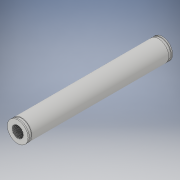
# Autodesk Inventor part: Axel_SBail
Saved by Autodesk Inventor 2019 (Build 230136000, 136)
## iProperties
Created: 2019-04-10
Part Number: Axel_SBail
Material: Generic
Document SubType Name: Modeling
Designer: samson.bailor
Density: 1 g/cm^3
Appearance: Default
Author: samson.bailor
Autodesk Inventor part; units mm, degrees
ref_plane "YZ Plane" through (0, 0, 0) normal (1, 0, 0) x (0, 1, 0)
ref_plane "XZ Plane" through (0, 0, 0) normal (0, 1, 0) x (-1, 0, 0)
ref_plane "XY Plane" through (0, 0, 0) normal (0, 0, 1) x (1, 0, 0)
sketch "Sketch1" plane through (0, 0, 0) normal (0, 0, 1) x (1, 0, 0)
  circle A0 centre (0, 0) radius 25.4
  dimension "d0" = 50.8
  constraints: 1 centre point, 1 coincident
  measures "d0" diameter of A0
extrude "Extrusion1" add sketch "Sketch1" along normal blind 355.6
sketch "Sketch2" plane through (0, 0, 355.6) normal (0, 0, 1) x (1, 0, 0)
  line L0 (0, 13.97) -> (0.508, 13.97)
  line L1 (0, 13.97) -> (-0.508, 13.97)
  line L2 (-0.508, 13.97) -> (-0.856, 12.6711)
  line L3 (-0.508, 13.97) -> (1.4308, 13.97) construction
  line L4 (0.508, 13.97) -> (0.856, 12.6711)
  line L5 (0.508, 13.97) -> (2.6446, 13.97) construction
  line L6 (-2.4076, 13.7703) -> (-1.7971, 12.5722)
  line L7 (-3.4014, 13.5591) -> (-3.4718, 12.2162)
  line L8 (-2.9045, 13.6647) -> (-3.4014, 13.5591)
  line L9 (-2.9045, 13.6647) -> (-2.4076, 13.7703)
  line L10 (-5.218, 12.9689) -> (-4.3718, 11.9238)
  line L11 (-6.1462, 12.5556) -> (-5.9358, 11.2275)
  line L12 (-5.6821, 12.7622) -> (-6.1462, 12.5556)
  line L13 (-5.6821, 12.7622) -> (-5.218, 12.9689)
  line L14 (-7.8004, 11.6006) -> (-6.7553, 10.7543)
  line L15 (-8.6223, 11.0034) -> (-8.1404, 9.748)
  line L16 (-8.2114, 11.302) -> (-8.6223, 11.0034)
  line L17 (-8.2114, 11.302) -> (-7.8004, 11.6006)
  line L18 (-10.0418, 9.7253) -> (-8.8437, 9.1148)
  line L19 (-10.7217, 8.9702) -> (-9.9893, 7.8425)
  line L20 (-10.3817, 9.3478) -> (-10.7217, 8.9702)
  line L21 (-10.3817, 9.3478) -> (-10.0418, 9.7253)
  line L22 (-11.8444, 7.4249) -> (-10.5455, 7.0769)
  line L23 (-12.3524, 6.5451) -> (-11.4015, 5.5942)
  line L24 (-12.0984, 6.985) -> (-12.3524, 6.5451)
  line L25 (-12.0984, 6.985) -> (-11.8444, 7.4249)
  line L26 (-13.1293, 4.8001) -> (-11.7864, 4.7297)
  line L27 (-13.4432, 3.8338) -> (-12.3155, 3.1015)
  line L28 (-13.2863, 4.317) -> (-13.4432, 3.8338)
  line L29 (-13.2863, 4.317) -> (-13.1293, 4.8001)
  line L30 (-13.8404, 1.9655) -> (-12.5122, 2.1758)
  line L31 (-13.9466, 0.955) -> (-12.6912, 0.4731)
  line L32 (-13.8935, 1.4603) -> (-13.9466, 0.955)
  line L33 (-13.8935, 1.4603) -> (-13.8404, 1.9655)
  line L34 (-13.9466, -0.955) -> (-12.6912, -0.4731)
  line L35 (-13.8404, -1.9655) -> (-12.5122, -2.1758)
  line L36 (-13.8935, -1.4603) -> (-13.8404, -1.9655)
  line L37 (-13.8935, -1.4603) -> (-13.9466, -0.955)
  line L38 (-13.4432, -3.8338) -> (-12.3155, -3.1015)
  line L39 (-13.1293, -4.8001) -> (-11.7864, -4.7297)
  line L40 (-13.2863, -4.317) -> (-13.1293, -4.8001)
  line L41 (-13.2863, -4.317) -> (-13.4432, -3.8338)
  line L42 (-12.3524, -6.5451) -> (-11.4015, -5.5942)
  line L43 (-11.8444, -7.4249) -> (-10.5455, -7.0769)
  line L44 (-12.0984, -6.985) -> (-11.8444, -7.4249)
  line L45 (-12.0984, -6.985) -> (-12.3524, -6.5451)
  line L46 (-10.7217, -8.9702) -> (-9.9893, -7.8425)
  line L47 (-10.0418, -9.7253) -> (-8.8437, -9.1148)
  line L48 (-10.3817, -9.3478) -> (-10.0418, -9.7253)
  line L49 (-10.3817, -9.3478) -> (-10.7217, -8.9702)
  line L50 (-8.6223, -11.0034) -> (-8.1404, -9.748)
  line L51 (-7.8004, -11.6006) -> (-6.7553, -10.7543)
  line L52 (-8.2114, -11.302) -> (-7.8004, -11.6006)
  line L53 (-8.2114, -11.302) -> (-8.6223, -11.0034)
  line L54 (-6.1462, -12.5556) -> (-5.9358, -11.2275)
  line L55 (-5.218, -12.9689) -> (-4.3718, -11.9238)
  line L56 (-5.6821, -12.7622) -> (-5.218, -12.9689)
  line L57 (-5.6821, -12.7622) -> (-6.1462, -12.5556)
  line L58 (-3.4014, -13.5591) -> (-3.4718, -12.2162)
  line L59 (-2.4076, -13.7703) -> (-1.7971, -12.5722)
  line L60 (-2.9045, -13.6647) -> (-2.4076, -13.7703)
  line L61 (-2.9045, -13.6647) -> (-3.4014, -13.5591)
  line L62 (-0.508, -13.97) -> (-0.856, -12.6711)
  line L63 (0.508, -13.97) -> (0.856, -12.6711)
  line L64 (0, -13.97) -> (0.508, -13.97)
  line L65 (0, -13.97) -> (-0.508, -13.97)
  line L66 (2.4076, -13.7703) -> (1.7971, -12.5722)
  line L67 (3.4014, -13.5591) -> (3.4718, -12.2162)
  line L68 (2.9045, -13.6647) -> (3.4014, -13.5591)
  line L69 (2.9045, -13.6647) -> (2.4076, -13.7703)
  line L70 (5.218, -12.9689) -> (4.3718, -11.9238)
  line L71 (6.1462, -12.5556) -> (5.9358, -11.2275)
  line L72 (5.6821, -12.7622) -> (6.1462, -12.5556)
  line L73 (5.6821, -12.7622) -> (5.218, -12.9689)
  line L74 (7.8004, -11.6006) -> (6.7553, -10.7543)
  line L75 (8.6223, -11.0034) -> (8.1404, -9.748)
  line L76 (8.2114, -11.302) -> (8.6223, -11.0034)
  line L77 (8.2114, -11.302) -> (7.8004, -11.6006)
  line L78 (10.0418, -9.7253) -> (8.8437, -9.1148)
  line L79 (10.7217, -8.9702) -> (9.9893, -7.8425)
  line L80 (10.3817, -9.3478) -> (10.7217, -8.9702)
  line L81 (10.3817, -9.3478) -> (10.0418, -9.7253)
  line L82 (11.8444, -7.4249) -> (10.5455, -7.0769)
  line L83 (12.3524, -6.5451) -> (11.4015, -5.5942)
  line L84 (12.0984, -6.985) -> (12.3524, -6.5451)
  line L85 (12.0984, -6.985) -> (11.8444, -7.4249)
  line L86 (13.1293, -4.8001) -> (11.7864, -4.7297)
  line L87 (13.4432, -3.8338) -> (12.3155, -3.1015)
  line L88 (13.2863, -4.317) -> (13.4432, -3.8338)
  line L89 (13.2863, -4.317) -> (13.1293, -4.8001)
  line L90 (13.8404, -1.9655) -> (12.5122, -2.1758)
  line L91 (13.9466, -0.955) -> (12.6912, -0.4731)
  line L92 (13.8935, -1.4603) -> (13.9466, -0.955)
  line L93 (13.8935, -1.4603) -> (13.8404, -1.9655)
  line L94 (13.9466, 0.955) -> (12.6912, 0.4731)
  line L95 (13.8404, 1.9655) -> (12.5122, 2.1758)
  line L96 (13.8935, 1.4603) -> (13.8404, 1.9655)
  line L97 (13.8935, 1.4603) -> (13.9466, 0.955)
  line L98 (13.4432, 3.8338) -> (12.3155, 3.1015)
  line L99 (13.1293, 4.8001) -> (11.7864, 4.7297)
  line L100 (13.2863, 4.317) -> (13.1293, 4.8001)
  line L101 (13.2863, 4.317) -> (13.4432, 3.8338)
  line L102 (12.3524, 6.5451) -> (11.4015, 5.5942)
  line L103 (11.8444, 7.4249) -> (10.5455, 7.0769)
  line L104 (12.0984, 6.985) -> (11.8444, 7.4249)
  line L105 (12.0984, 6.985) -> (12.3524, 6.5451)
  line L106 (10.7217, 8.9702) -> (9.9893, 7.8425)
  line L107 (10.0418, 9.7253) -> (8.8437, 9.1148)
  line L108 (10.3817, 9.3478) -> (10.0418, 9.7253)
  line L109 (10.3817, 9.3478) -> (10.7217, 8.9702)
  line L110 (8.6223, 11.0034) -> (8.1404, 9.748)
  line L111 (7.8004, 11.6006) -> (6.7553, 10.7543)
  line L112 (8.2114, 11.302) -> (7.8004, 11.6006)
  line L113 (8.2114, 11.302) -> (8.6223, 11.0034)
  line L114 (6.1462, 12.5556) -> (5.9358, 11.2275)
  line L115 (5.218, 12.9689) -> (4.3718, 11.9238)
  line L116 (5.6821, 12.7622) -> (5.218, 12.9689)
  line L117 (5.6821, 12.7622) -> (6.1462, 12.5556)
  line L118 (3.4014, 13.5591) -> (3.4718, 12.2162)
  line L119 (2.4076, 13.7703) -> (1.7971, 12.5722)
  line L120 (2.9045, 13.6647) -> (2.4076, 13.7703)
  line L121 (2.9045, 13.6647) -> (3.4014, 13.5591)
  arc A0 (-0.856, 12.6711) -> (-1.7971, 12.5722) centre (0, 0) ccw
  arc A1 (1.7971, 12.5722) -> (0.856, 12.6711) centre (0, 0) ccw
  arc A2 (4.3718, 11.9238) -> (3.4718, 12.2162) centre (0, 0) ccw
  arc A3 (6.7553, 10.7543) -> (5.9358, 11.2275) centre (0, 0) ccw
  arc A4 (8.8437, 9.1148) -> (8.1404, 9.748) centre (0, 0) ccw
  arc A5 (10.5455, 7.0769) -> (9.9893, 7.8425) centre (0, 0) ccw
  arc A6 (11.7864, 4.7297) -> (11.4015, 5.5942) centre (0, 0) ccw
  arc A7 (12.5122, 2.1758) -> (12.3155, 3.1015) centre (0, 0) ccw
  arc A8 (12.6912, -0.4731) -> (12.6912, 0.4731) centre (0, 0) ccw
  arc A9 (12.3155, -3.1015) -> (12.5122, -2.1758) centre (0, 0) ccw
  arc A10 (11.4015, -5.5942) -> (11.7864, -4.7297) centre (0, 0) ccw
  arc A11 (9.9893, -7.8425) -> (10.5455, -7.0769) centre (0, 0) ccw
  arc A12 (8.1404, -9.748) -> (8.8437, -9.1148) centre (0, 0) ccw
  arc A13 (5.9358, -11.2275) -> (6.7553, -10.7543) centre (0, 0) ccw
  arc A14 (3.4718, -12.2162) -> (4.3718, -11.9238) centre (0, 0) ccw
  arc A15 (0.856, -12.6711) -> (1.7971, -12.5722) centre (0, 0) ccw
  arc A16 (-1.7971, -12.5722) -> (-0.856, -12.6711) centre (0, 0) ccw
  arc A17 (-4.3718, -11.9238) -> (-3.4718, -12.2162) centre (0, 0) ccw
  arc A18 (-6.7553, -10.7543) -> (-5.9358, -11.2275) centre (0, 0) ccw
  arc A19 (-8.8437, -9.1148) -> (-8.1404, -9.748) centre (0, 0) ccw
  arc A20 (-10.5455, -7.0769) -> (-9.9893, -7.8425) centre (0, 0) ccw
  arc A21 (-11.7864, -4.7297) -> (-11.4015, -5.5942) centre (0, 0) ccw
  arc A22 (-12.5122, -2.1758) -> (-12.3155, -3.1015) centre (0, 0) ccw
  arc A23 (-12.6912, 0.4731) -> (-12.6912, -0.4731) centre (0, 0) ccw
  arc A24 (-12.3155, 3.1015) -> (-12.5122, 2.1758) centre (0, 0) ccw
  arc A25 (-11.4015, 5.5942) -> (-11.7864, 4.7297) centre (0, 0) ccw
  arc A26 (-9.9893, 7.8425) -> (-10.5455, 7.0769) centre (0, 0) ccw
  arc A27 (-8.1404, 9.748) -> (-8.8437, 9.1148) centre (0, 0) ccw
  arc A28 (-3.4718, 12.2162) -> (-4.3718, 11.9238) centre (0, 0) ccw
  arc A29 (-5.9358, 11.2275) -> (-6.7553, 10.7543) centre (0, 0) ccw
  dimension "d5" = 0.508
  dimension "d6" = 0.508
  dimension "d7" = 105
  dimension "d8" = 75
  dimension "d11" = 360
  constraints: 244 end point, 120 equal length, 4 horizontal, 4 vertical alignment, 237 other
  measures "d5" distance of L0.start L0.end
  measures "d6" distance of L0.start L1.end
  measures "d7" angle of L2 L3
  measures "d8" angle of L4 L5
extrude "Extrusion2" cut sketch "Sketch2" against normal through all
sketch "Sketch3" plane through (0, 0, 0) normal (0, 0, -1) x (-1, 0, 0)
  line L0 (11.7864, -4.7297) -> (13.1293, -4.8001) projected
  circle A0 centre (0, 0) radius 13.9792
  constraints: 1 coincident, 3 other
extrude "Extrusion3" cut sketch "Sketch3" against normal blind 330.2
sketch "Sketch4" plane through (0, 0, 355.6) normal (0, 0, 1) x (1, 0, 0)
  line L0 (31.0854, 16.4706) -> (47.788, 16.4706)
  line L1 (47.788, 16.4706) -> (47.788, 0)
  line L2 (47.788, 0) -> (31.0854, 0)
  line L3 (31.0854, 0) -> (31.0854, 16.4706)
  point P0 (0, 0)
  constraints: 8 end point, 2 parallel, 1 horizontal, 1 perpendicular
extrude "Extrusion4" add sketch "Sketch4" against normal blind 3.175
sketch "Sketch5" plane through (0, 0, 352.425) normal (0, 0, -1) x (-1, 0, 0)
  circle A0 centre (0, 0) radius 25.4
  circle A1 centre (0, 0) radius 23.8125
  dimension "d19" = 1.5875
  constraints: 2 centre point, 1 coincident
  measures "d19" radial gap between concentric circles of A0 A1
extrude "Extrusion5" cut sketch "Sketch5" along normal blind 6.35
sketch "Sketch6" plane through (0, 0, 0) normal (0, 0, -1) x (-1, 0, 0)
  line L0 (29.0417, -43.641) -> (10.5178, -43.641)
  line L1 (10.5178, -43.641) -> (10.5178, -69.3861)
  line L2 (10.5178, -69.3861) -> (29.0417, -69.3861)
  line L3 (29.0417, -69.3861) -> (29.0417, -43.641)
  point P0 (0, 0)
  constraints: 8 end point, 2 parallel, 1 horizontal, 1 perpendicular
extrude "Extrusion6" add sketch "Sketch6" against normal blind 3.175
sketch "Sketch7" plane through (0, 0, 3.175) normal (0, 0, 1) x (1, 0, 0)
  circle A0 centre (0, 0) radius 25.4
  circle A1 centre (0, 0) radius 23.8125
  constraints: 2 centre point, 2 coincident
extrude "Extrusion7" cut sketch "Sketch7" along normal blind 6.35
sketch "Sketch8" plane through (-29.0417, -69.3861, 0) normal (-1, 0, 0) x (0, 0, 1)
  line L0 (0, 0) -> (0, 25.7451) projected
  line L1 (3.175, 25.7451) -> (3.175, 0) projected
  line L2 (0, 0) -> (3.175, 0)
  line L3 (3.175, 0) -> (3.175, 25.7451)
  line L4 (3.175, 25.7451) -> (0, 25.7451)
  line L5 (0, 25.7451) -> (0, 0)
  point P0 (0, 69.3861)
  constraints: 8 end point, 2 parallel, 1 horizontal, 1 perpendicular
extrude "Extrusion8" cut sketch "Sketch8" against normal through all
sketch "Sketch9" plane through (0, 0, 355.6) normal (0, 0, 1) x (1, 0, 0)
  line L0 (31.0854, 16.4706) -> (47.788, 16.4706) projected
  line L1 (31.0854, 16.4706) -> (47.788, 16.4706)
  line L2 (47.788, 16.4706) -> (47.788, 0)
  line L3 (47.788, 0) -> (31.0854, 0)
  line L4 (31.0854, 0) -> (31.0854, 16.4706)
  point P0 (0, 0)
  constraints: 8 end point, 2 parallel, 1 horizontal, 1 perpendicular
extrude "Extrusion9" cut sketch "Sketch9" against normal blind 6.35
body "Solid1"
